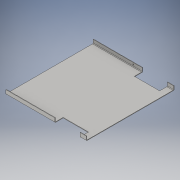
# Autodesk Inventor part: BellyPan2
Saved by Autodesk Inventor 2016 (Build 200138000, 138)
## iProperties
Created: 2017-01-21
Part Number: BellyPan2
Material: Generic
Document SubType Name: Modeling
Designer: hamblettk
Density: 1 g/cm^3
Appearance: Default
Author: hamblettk
Autodesk Inventor part; units mm, degrees
ref_plane "YZ Plane" through (0, 0, 0) normal (1, 0, 0) x (0, 1, 0)
ref_plane "XZ Plane" through (0, 0, 0) normal (0, 1, 0) x (-1, 0, 0)
ref_plane "XY Plane" through (0, 0, 0) normal (0, 0, 1) x (1, 0, 0)
sketch "Sketch1" plane through (0, 0, 0) normal (0, 1, 0) x (-1, 0, 0)
  line L0 (0, 0) -> (495.3, 0)
  line L1 (495.3, 0) -> (495.3, -539.75)
  line L2 (495.3, -539.75) -> (0, -539.75)
  line L3 (0, -539.75) -> (0, 0)
  dimension "d0" = 495.3
  dimension "d1" = 539.75
  constraints: 8 end point, 2 parallel, 1 horizontal, 1 perpendicular
  measures "d0" distance of L1.end L2.end
  measures "d1" distance of L0.end L1.end
extrude "Extrusion1" add sketch "Sketch1" along normal blind 3.175
sketch "Sketch2" plane through (0, 0, 0) normal (1, 0, 0) x (0, 0, -1)
  line L0 (0, 3.175) -> (0, 15.875)
  line L1 (0, 15.875) -> (3.175, 15.875)
  line L2 (3.175, 15.875) -> (3.175, 3.175)
  line L3 (0, 3.175) -> (539.75, 3.175) projected
  line L4 (3.175, 3.175) -> (0, 3.175)
  line L5 (539.75, 3.175) -> (539.75, 15.875)
  line L6 (539.75, 15.875) -> (536.575, 15.875)
  line L7 (536.575, 15.875) -> (536.575, 3.175)
  line L8 (539.75, 0) -> (539.75, 3.175) projected
  line L9 (536.575, 3.175) -> (539.75, 3.175)
  point P0 (0, 0)
  dimension "d4" = 12.7
  dimension "d5" = 3.175
  dimension "d6" = 12.7
  dimension "d7" = 3.175
  constraints: 16 end point, 5 perpendicular, 2 vertical, 1 horizontal, 1 point on line
  measures "d4" distance of L0.start L0.end
  measures "d5" distance of L0.end L1.end
  measures "d6" distance of L3.end L5.end
  measures "d7" distance of L5.end L6.end
extrude "Extrusion2" add sketch "Sketch2" against normal blind 495.3
fillet "Fillet1" radius 3.175 4 edges at (-247.65, 3.175, -536.575) (-247.65, 3.175, -3.175) (-247.65, 0, 0) (-247.65, 0, -539.75)
sketch "Sketch3" plane through (-495.3, 15.875, -539.75) normal (0, 1, 0) x (1, 0, 0)
  line L0 (495.3, 0) -> (0, 0) projected
  line L1 (495.3, 0) -> (457.2, 0)
  line L2 (457.2, 0) -> (304.8, 0)
  line L3 (304.8, 0) -> (304.8, -50.8)
  line L4 (304.8, -50.8) -> (457.2, -50.8)
  line L5 (457.2, -50.8) -> (457.2, 0)
  line L6 (0, -6.35) -> (0, -533.4) projected
  line L7 (0, -269.875) -> (495.3, -269.875)
  line L8 (495.3, -539.75) -> (0, -539.75)
  line L9 (457.2, -539.75) -> (304.8, -539.75)
  line L10 (304.8, -539.75) -> (304.8, -488.95)
  line L11 (304.8, -488.95) -> (457.2, -488.95)
  line L12 (457.2, -488.95) -> (457.2, -539.75)
  point P0 (495.3, -539.75)
  dimension "d11" = 38.1
  dimension "d12" = 152.4
  dimension "d13" = 50.8
  constraints: 22 end point, 6 symmetric about line, 4 point on line, 2 horizontal, 1 midpoint, 1 perpendicular, 1 vertical
  measures "d11" distance of L0.start L1.end
  measures "d12" distance of L1.end L2.end
  measures "d13" distance of L2.end L3.end
extrude "Extrusion3" cut sketch "Sketch3" against normal blind 495.3
sketch "Sketch5" plane through (-495.3, 15.875, -3.175) normal (0, 1, 0) x (1, 0, 0)
  line L0 (304.8, -3.175) -> (304.8, 0) projected
  line L1 (304.8, 0) -> (0, 0) projected
  line L2 (0, -3.175) -> (0, 0) projected
  line L3 (304.8, -3.175) -> (0, -3.175) projected
  line L4 (457.2, 0) -> (457.2, -3.175) projected
  line L5 (495.3, -3.175) -> (457.2, -3.175) projected
  line L6 (495.3, 0) -> (495.3, -3.175) projected
  line L7 (495.3, 0) -> (457.2, 0) projected
  line L8 (457.2, 536.575) -> (457.2, 533.4) projected
  line L9 (495.3, 533.4) -> (457.2, 533.4) projected
  line L10 (495.3, 536.575) -> (495.3, 533.4) projected
  line L11 (495.3, 536.575) -> (457.2, 536.575) projected
  line L12 (304.8, 533.4) -> (304.8, 536.575) projected
  line L13 (304.8, 536.575) -> (0, 536.575) projected
  line L14 (0, 533.4) -> (0, 536.575) projected
  line L15 (304.8, 533.4) -> (0, 533.4) projected
extrude "Extrusion4" add sketch "Sketch5" along normal blind 9.525
sketch "Sketch6" plane through (-190.5, 0, -50.8) normal (1, 0, 0) x (0, 0, -1)
  line L0 (0, 0) -> (-47.625, 0) projected
  line L1 (0, 3.175) -> (0, 0) projected
  line L2 (-44.45, 3.175) -> (0, 3.175) projected
  arc A0 (-47.625, 6.35) -> (-44.45, 3.175) centre (-44.45, 6.35) ccw projected
  line L3 (-47.625, 25.4) -> (-47.625, 6.35) projected
  line L4 (-50.8, 25.4) -> (-47.625, 25.4) projected
  line L5 (-50.8, 3.175) -> (-50.8, 25.4) projected
  arc A1 (-50.8, 3.175) -> (-47.625, 0) centre (-47.625, 3.175) ccw projected
  line L6 (485.775, 0) -> (438.15, 0) projected
  arc A2 (485.775, 0) -> (488.95, 3.175) centre (485.775, 3.175) ccw projected
  line L7 (488.95, 25.4) -> (488.95, 3.175) projected
  line L8 (485.775, 25.4) -> (488.95, 25.4) projected
  line L9 (485.775, 6.35) -> (485.775, 25.4) projected
  arc A3 (482.6, 3.175) -> (485.775, 6.35) centre (482.6, 6.35) ccw projected
  line L10 (438.15, 3.175) -> (482.6, 3.175) projected
  line L11 (438.15, 3.175) -> (438.15, 0) projected
  point P0 (-50.8, 0)
extrude "Extrusion5" cut sketch "Sketch6" against normal blind 3.175
sketch "Sketch7" plane through (-495.3, 6.35, -536.575) normal (0, 0, 1) x (1, 0, 0)
  line L0 (301.625, 0) -> (301.625, 19.05) projected
  line L1 (301.625, 9.525) -> (247.65, 9.525)
  circle A0 centre (247.65, 9.525) radius 3.5687
  point P0 (495.3, -6.35)
  dimension "d21" = 7.1374
  dimension "d22" = 53.975
  constraints: 2 end point, 1 centre point, 1 coincident, 1 horizontal, 1 midpoint
  measures "d21" diameter of A0
  measures "d22" distance from line of L0 L1.end
extrude "Extrusion6" cut sketch "Sketch7" against normal blind 3.175
body "Solid1"
